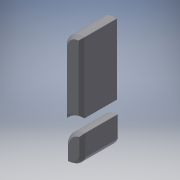
# Autodesk Inventor part: literai
Saved by Autodesk Inventor 2019 (Build 230136000, 136)
## iProperties
Created: 2020-10-14
Part Number: literai
Material: Ogólny
Document SubType Name: Modeling
Designer: Dawid
Density: 1 g/cm^3
Appearance: Domyślna
Author: Dawid
Autodesk Inventor part; units mm, degrees
ref_plane "YZ Plane" through (0, 0, 0) normal (1, 0, 0) x (0, 1, 0)
ref_plane "XZ Plane" through (0, 0, 0) normal (0, 1, 0) x (-1, 0, 0)
ref_plane "XY Plane" through (0, 0, 0) normal (0, 0, 1) x (1, 0, 0)
sketch "Szkic1" plane through (0, 0, 0) normal (0, 0, 1) x (1, 0, 0)
  line L0 (-1.3108, -12.905) -> (-1.3108, -10.0385)
  spline S0 degree 4 poles (1.6306, -10.8768) (1.5249, -11.1473) (1.3425, -11.497) (1.0422, -11.89) (0.5755, -12.2734) (0.0272, -12.6005) (-0.5028, -12.7796) (-0.9603, -12.8671) (-1.3108, -12.905) knots 0 0 0 0 0 0.304305 0.424541 0.545967 0.670392 1 1 1 1 1
  line L1 (1.6306, -7.3073) -> (1.6306, -10.8768)
  spline S1 degree 4 poles (-1.3108, -10.0385) (-1.206, -9.6395) (-1.0239, -9.1317) (-0.7187, -8.5698) (-0.2302, -8.04) (0.3127, -7.6275) (0.838, -7.4177) (1.2888, -7.3323) (1.6306, -7.3073) knots 0 0 0 0 0 0.330819 0.454349 0.5746 0.693981 1 1 1 1 1
  line L2 (1.4656, 6.6497) -> (1.4656, -5.2511)
  spline S2 degree 4 poles (-1.4677, 4.5193) (-1.3642, 4.8752) (-1.1849, 5.3226) (-0.8831, 5.8051) (-0.4003, 6.232) (0.1453, 6.5459) (0.6724, 6.6654) (1.1231, 6.6778) (1.4656, 6.6497) knots 0 0 0 0 0 0.32512 0.446527 0.565537 0.685202 1 1 1 1 1
  line L3 (-1.4677, -6.633) -> (-1.4677, 4.5193)
  spline S3 degree 4 poles (1.4656, -5.2511) (1.2149, -5.2472) (0.8691, -5.2729) (0.4353, -5.3641) (-0.0733, -5.5664) (-0.5802, -5.8367) (-0.973, -6.1352) (-1.2651, -6.4124) (-1.4677, -6.633) knots 0 0 0 0 0 0.303835 0.42546 0.548402 0.673696 1 1 1 1 1
  point P0 (0, 0)
  point P1 (-1.1027, -9.3964)
  point P2 (-0.8481, -8.8578)
  point P3 (-0.5505, -8.4115)
  point P4 (-0.2114, -8.0475)
  point P5 (0.171, -7.7579)
  point P6 (0.6007, -7.5381)
  point P7 (1.0846, -7.387)
  point P8 (1.4326, -11.2981)
  point P9 (1.1911, -11.6655)
  point P10 (0.9057, -11.9842)
  point P11 (0.5741, -12.2575)
  point P12 (0.1924, -12.4873)
  point P13 (-0.2447, -12.6734)
  point P14 (-0.7436, -12.8138)
  point P15 (-1.2615, 5.0896)
  point P16 (-1.0108, 5.5545)
  point P17 (-0.7192, 5.9272)
  point P18 (-0.3866, 6.2187)
  point P19 (-0.0096, 6.4362)
  point P20 (0.4186, 6.5827)
  point P21 (0.9069, 6.656)
  point P22 (1.0656, -5.2667)
  point P23 (0.6788, -5.3253)
  point P24 (0.303, -5.427)
  point P25 (-0.0637, -5.5723)
  point P26 (-0.423, -5.7628)
  point P27 (-0.7762, -6.001)
  point P28 (-1.1243, -6.2899)
  constraints: 8 end point, 36 other
extrude "Wyciągnięcie proste1" add sketch "Szkic1" along normal blind 6
chamfer "Faza1" distance 0.5 angle 45 8 edges at (-1.3108, -11.4717, 6) (-0.2598, -8.0923, 6) (1.6306, -9.0921, 6) (0.5252, -12.2913, 6) (-0.1065, -5.5924, 6) (-1.4677, -1.0569, 6) (-0.4068, 6.204, 6) (1.4656, 0.6993, 6)
